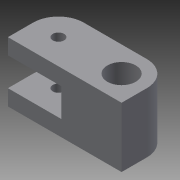
# Autodesk Inventor part: Y-idler
Saved by Autodesk Inventor 2015 (Build 190159000, 159)
## iProperties
Created: 2015-04-28
Part Number: Y-idler
Material: Generic
Document SubType Name: Modeling
Designer: X
Density: 1 g/cm^3
Appearance: Default
Author: X
Autodesk Inventor part; units mm, degrees
ref_plane "YZ Plane" through (0, 0, 0) normal (1, 0, 0) x (0, 1, 0)
ref_plane "XZ Plane" through (0, 0, 0) normal (0, 1, 0) x (-1, 0, 0)
sketch "Sketch1" plane through (0, 0, 0) normal (0, 0, 1) x (1, 0, 0)
  circle A0 centre (0, 0) radius 8
  circle A1 centre (20, 0) radius 8
  line L0 (0, 8) -> (20, 8)
  line L1 (-8, -8) -> (28, -8)
  line L2 (28, 0) -> (28, -8)
  line L3 (-8, 0) -> (-8, -8)
  dimension "d0" = 16
  dimension "d2" = 36
  constraints: 8 end point, 5 tangent, 4 point on circle, 3 coincident, 2 centre point, 2 perpendicular, 1 equal radius, 1 horizontal, 1 parallel
  measures "d0" diameter of A0
  measures "d2" distance of L1.start L1.end
extrude "Extrusion1" add sketch "Sketch1" along normal blind 19
sketch "Sketch2" plane through (0, 0, 0) normal (0, 0, -1) x (-1, 0, 0)
  line L0 (-20, 8) -> (0, 8) projected
  line L1 (8, 0) -> (8, -8) projected
  line L2 (-28, -8) -> (-28, 0) projected
  point P0 (0, 0)
  point P1 (0, 0)
  dimension "d5" = 8
  dimension "d6" = 8
  measures "d5" distance from line of L0 point (0, 0)
  measures "d6" distance from line of L1 point (0, 0)
hole "Hole1" at (0, 0, 0) direction (0, 0, 1) diameter 3.6 end through all
sketch "Sketch3" plane through (0, 0, 0) normal (0, 0, -1) x (-1, 0, 0)
  line L0 (-28, -8) -> (-28, 0) projected
  line L1 (-20, 8) -> (0, 8) projected
  point P0 (0, 0)
  point P1 (-20, 0)
  dimension "d16" = 8
  dimension "d17" = 8
  measures "d16" distance from line of point (-20, 0) L0
  measures "d17" distance from line of L1 point (-20, 0)
hole "Hole2" at (20, 0, 0) direction (0, 0, 1) diameter 9 end through all
ref_plane "Work Plane1" through (0, 0, 0) normal (0, 1, 0) x (1, 0, 0)
sketch "Sketch7" plane through (0, 0, 0) normal (0, 1, 0) x (1, 0, 0)
  line L0 (12, -5) -> (0, -5)
  line L1 (0, -5) -> (0, -14)
  line L2 (0, -14) -> (12, -14)
  line L3 (12, -14) -> (12, -5)
  line L4 (12, -5) -> (0, -14) construction
  line L5 (0, -5) -> (12, -14) construction
  line L6 (0, 0) -> (0, -19) projected
  line L7 (-8, -19) -> (0, -19) projected
  line L8 (20, -19) -> (0, -19) projected
  line L9 (0, -22.8) -> (0, 3.8) projected
  point P0 (6, -9.5)
  dimension "d32" = 12
  dimension "d34" = 9.5
  dimension "d35" = 9
  constraints: 12 end point, 2 midpoint, 2 parallel, 1 horizontal, 1 perpendicular, 1 point on line
  measures "d32" distance of L1.end L2.end
  measures "d34" distance from line of L8 point (6, -9.5)
  measures "d35" distance of L0.end L1.end
revolve "Revolution2" cut sketch "Sketch7" angle 360 about axis through (0, 0, 43.7379) along (0, 0, -1)
equation "\"d5\" = 0.5 * d0"
equation "\"d6\" = 0.5 * d0"
equation "\"d16\" = 0.5 * d0"
equation "\"d17\" = 0.5 * d0"
equation "\"d34\" = 0.5 * d3"
equation "\"d3\" = 19"
body "Solid1"
